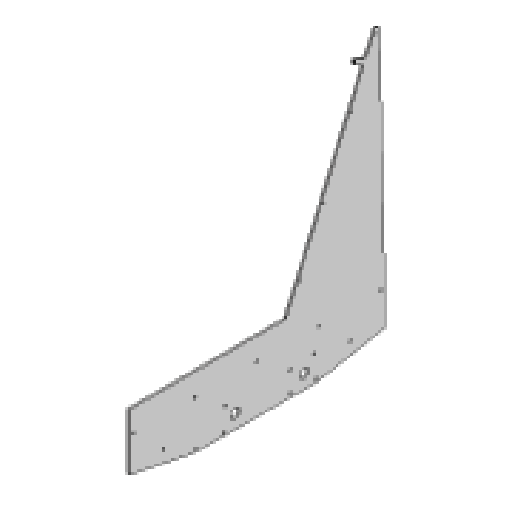
# Autodesk Inventor part: Outside Chassi Plate low 2.0
Saved by Autodesk Inventor 2023 (Build 270158000, 158)
## iProperties
Created: 2022-09-05
Part Number: Outside Chassi Plate low 2.0
Material: Generic
Document SubType Name: Modeling
Designer: deli
Density: 1 g/cm^3
Appearance: Default
Author: deli
Autodesk Inventor part; units mm, degrees
ref_plane "YZ Plane" through (0, 0, 0) normal (1, 0, 0) x (0, 1, 0)
ref_plane "XZ Plane" through (0, 0, 0) normal (0, 1, 0) x (-1, 0, 0)
ref_plane "XY Plane" through (0, 0, 0) normal (0, 0, 1) x (1, 0, 0)
sketch "Sketch1" plane through (0, 0, 0) normal (1, 0, 0) x (0, 1, 0)
  line L0 (-213.0456, 518.5703) -> (-297.1987, 518.5703)
  line L1 (-297.1987, 518.5703) -> (-316.9444, 421.9583)
  line L2 (-213.7388, 140.8703) -> (-297.8918, 140.8703)
  circle A0 centre (-289.0456, 468.5703) radius 2
  circle A1 centre (-289.0456, 468.5703) radius 48 construction
  arc A2 (-277.131, 467.8463) -> (-300.9481, 469.4724) centre (-289.0456, 468.5703) ccw construction
  circle A3 centre (-289.0456, 190.8703) radius 48 construction
  arc A4 (-300.901, 189.4801) -> (-277.1614, 191.9869) centre (-289.0456, 190.8703) ccw construction
  circle A5 centre (-289.0456, 190.8703) radius 2
  circle A6 centre (-296.2956, 362.3801) radius 7
  circle A7 centre (-296.2956, 259.5275) radius 7
  circle A8 centre (-296.2956, 362.3801) radius 18.75 construction
  circle A9 centre (-296.2956, 259.5275) radius 18.75 construction
  arc A10 (-308.9916, 363.3423) -> (-283.5867, 361.6078) centre (-296.2956, 362.3801) ccw construction
  arc A11 (-283.6191, 260.7186) -> (-308.9414, 258.0446) centre (-296.2956, 259.5275) ccw construction
  line L3 (-277.131, 467.8463) -> (-283.5867, 361.6078) construction
  line L4 (-308.9916, 363.3423) -> (-300.9481, 469.4724) construction
  line L5 (-283.6191, 260.7186) -> (-277.1614, 191.9869) construction
  line L6 (-300.901, 189.4801) -> (-308.9414, 258.0446) construction
  circle A12 centre (-281.2909, 280.4541) radius 2
  circle A13 centre (-311.3004, 280.4541) radius 2
  circle A14 centre (-312.0456, 379.4828) radius 2
  circle A15 centre (-312.0456, 242.4249) radius 2
  circle A16 centre (-278.1266, 245.0207) radius 2
  circle A17 centre (-246.0456, 513.5703) radius 2
  arc A18 (-317.0456, 229.9036) -> (-317.0456, 229.9036) centre (-294.2956, 229.9036) ccw
  line L7 (-317.0456, 242.4249) -> (-317.0456, 229.9036)
  arc A19 (-316.9444, 421.9583) -> (-317.0456, 420.9571) centre (-312.0456, 420.9571) ccw
  line L8 (-317.0456, 420.9571) -> (-317.0456, 229.9036)
  line L9 (-297.8918, 140.8703) -> (-316.9582, 241.4941)
  circle A20 centre (-278.6149, 377.4783) radius 2
  arc A21 (-317.0456, 242.4249) -> (-316.9582, 241.4941) centre (-312.0456, 242.4249) ccw
  circle A22 centre (-246.0456, 237.7953) radius 2
  line L10 (-213.0456, 518.5703) -> (-213.0456, 285.8158)
  circle A23 centre (-246.0456, 421.6453) radius 2
  circle A24 centre (-246.0456, 329.7203) radius 2
  circle A25 centre (-312.0456, 420.9571) radius 2
  circle A26 centre (-246.0456, 145.8703) radius 2
  line L11 (-179.9838, 271.6186) -> (-182.7458, 265.1866)
  line L12 (-182.7458, 265.1866) -> (92.9136, 146.8149)
  line L13 (92.9136, 146.8149) -> (95.6756, 153.2469)
  line L14 (628.6384, -183.2052) -> (619.1262, -197.2948) construction
  line L15 (-182.3379, 278.8085) -> (-189.0456, 263.1877) construction
  line L16 (-188.4024, 281.4126) -> (108.5747, 153.8869) construction
  line L17 (102.5102, 156.491) -> (95.8025, 140.8703) construction
  line L18 (95.8025, 140.8703) -> (-189.0456, 263.1877) construction
  line L19 (-184.6634, 286.0648) -> (-173.6371, 281.3299) construction
  line L20 (-173.6371, 281.3299) -> (-175.2154, 277.6545) construction
  line L21 (-175.2154, 277.6545) -> (-186.2417, 282.3893) construction
  line L22 (-186.2417, 282.3893) -> (-184.6634, 286.0648) construction
  line L23 (-185.4431, 288.3041) -> (-176.0707, 284.2795) construction
  line L24 (-178.4381, 278.7663) -> (-187.8106, 282.7909) construction
  line L25 (-176.0707, 284.2795) -> (-176.6626, 282.9012) construction
  line L26 (-178.4381, 278.7663) -> (-179.03, 277.388) construction
  line L27 (-176.6626, 282.9012) -> (-186.035, 286.9258) construction
  arc A27 (-185.4431, 288.3041) -> (-188.4024, 281.4126) centre (-186.9228, 284.8584) ccw construction
  arc A28 (-186.035, 286.9258) -> (-187.8106, 282.7909) centre (-186.9228, 284.8584) ccw construction
  line L28 (99.2023, 157.9115) -> (99.7941, 159.2898) construction
  line L29 (99.7941, 159.2898) -> (109.1666, 155.2652) construction
  arc A29 (109.1666, 155.2652) -> (110.9421, 159.4) centre (110.0544, 157.3326) ccw construction
  line L30 (110.9421, 159.4) -> (101.5697, 163.4247) construction
  line L31 (101.5697, 163.4247) -> (102.1616, 164.803) construction
  line L32 (102.1616, 164.803) -> (111.534, 160.7783) construction
  arc A30 (108.5747, 153.8869) -> (111.534, 160.7783) centre (110.0544, 157.3326) ccw construction
  line L33 (109.3733, 159.8016) -> (107.795, 156.1262) construction
  line L34 (107.795, 156.1262) -> (96.7686, 160.8611) construction
  line L35 (96.7686, 160.8611) -> (98.3469, 164.5365) construction
  line L36 (98.3469, 164.5365) -> (109.3733, 159.8016) construction
  line L37 (92.9136, 146.8149) -> (-213.7388, 140.8703)
  circle A31 centre (-174.4733, 265.4433) radius 1
  circle A32 centre (-91.7755, 229.9318) radius 1
  circle A33 centre (4.7053, 188.5017) radius 1
  circle A34 centre (87.4031, 152.9902) radius 1
  circle A35 centre (73.8024, 178.3411) radius 1.5
  arc A36 (76.559, 177.1574) -> (71.0458, 179.5248) centre (73.8024, 178.3411) ccw
  line L38 (71.0458, 179.5248) -> (67.2322, 170.6439)
  line L39 (76.559, 177.1574) -> (72.7454, 168.2765)
  line L40 (95.6756, 153.2469) -> (75.2424, 162.0212)
  line L41 (60.977, 168.147) -> (-213.0456, 285.8158)
  arc A37 (72.7454, 168.2765) -> (75.2424, 162.0212) centre (77.1215, 166.3973) ccw
  arc A38 (60.977, 168.147) -> (67.2322, 170.6439) centre (62.8562, 172.523) ccw
  circle A39 centre (73.8024, 178.3411) radius 6 construction
  circle A40 centre (-215.5456, 495.2703) radius 1.6
  circle A41 centre (-230.5456, 495.2703) radius 1.6
  circle A42 centre (-230.5456, 485.2703) radius 1.6
  circle A43 centre (-215.5456, 485.2703) radius 1.6
  circle A44 centre (-215.5456, 466.3703) radius 1.6
  circle A45 centre (-215.5456, 456.3703) radius 1.6
  circle A46 centre (-230.5456, 456.3703) radius 1.6
  circle A47 centre (-230.5456, 466.3703) radius 1.6
  line L42 (-215.5456, 495.2703) -> (-230.5456, 495.2703) construction
  line L43 (-230.5456, 495.2703) -> (-230.5456, 485.2703) construction
  line L44 (-230.5456, 485.2703) -> (-215.5456, 485.2703) construction
  line L45 (-215.5456, 485.2703) -> (-215.5456, 495.2703) construction
  line L46 (-215.5456, 456.3703) -> (-215.5456, 466.3703) construction
  line L47 (-215.5456, 466.3703) -> (-230.5456, 466.3703) construction
  line L48 (-230.5456, 466.3703) -> (-230.5456, 456.3703) construction
  line L49 (-230.5456, 456.3703) -> (-215.5456, 456.3703) construction
  point P0 (0, 0)
  point P1 (-317.0456, 242.4249)
  point P2 (-225.2933, 140.8703)
  dimension "d44" = 4
  dimension "d46" = 96
  dimension "d47" = 23.8732
  dimension "d48" = 96
  dimension "d49" = 4
  dimension "d51" = 23.8732
  dimension "d54" = 50
  dimension "d55" = 50
  dimension "d58" = 14
  dimension "d59" = 14
  dimension "d60" = 37.5
  dimension "d61" = 37.5
  dimension "d62" = 25.4648
  dimension "d63" = 25.4648
  dimension "d64" = 179.143
  dimension "d65" = 179.143
  dimension "d66" = 178.679
  dimension "d67" = 178.679
  dimension "d68" = 106.4344
  dimension "d70" = 69.0344
  dimension "d74" = 4
  dimension "d75" = 4
  dimension "d77" = 4
  dimension "d78" = 4
  dimension "d94" = 2.5
  dimension "d95" = 2.5
  dimension "d97" = 2.5
  dimension "d103" = 4
  dimension "d120" = 4
  dimension "d124" = 28
  dimension "d125" = 20.75
  dimension "d127" = 20.75
  dimension "d142" = 4
  dimension "d143" = 2.5
  dimension "d144" = 4
  dimension "d145" = 4
  dimension "d146" = 18
  dimension "d147" = 18
  dimension "d148" = 5
  dimension "d149" = 5
  dimension "d153" = 4
  dimension "d166" = 5
  dimension "d218" = 0
  dimension "d235" = 33
  dimension "d244" = 28
  dimension "d246" = 84.153
  dimension "d247" = 84.153
  dimension "d258" = 5
  dimension "d259" = 5
  dimension "d260" = 4
  dimension "d261" = 4
  dimension "d262" = 4
  dimension "d264" = 5
  dimension "d266" = 33
  dimension "d267" = 33
  dimension "d268" = 91.925
  dimension "d269" = 91.925
  dimension "d270" = 91.925
  dimension "d271" = 0
  dimension "d272" = 41.4743
  dimension "d277" = 5
  dimension "d296" = 33
  dimension "d297" = 7
  dimension "d317" = 0
  constraints: 100 end point, 48 centre point, 29 point on circle, 28 tangent, 23 perpendicular, 15 parallel, 12 equal radius, 10 coincident, 7 point on line, 4 collinear, 4 vertical, 3 concentric, 3 equal length
  measures "d44" diameter of A0
  measures "d46" diameter of A1
  measures "d47" diameter of A2
  measures "d48" diameter of A3
  measures "d49" diameter of A5
  measures "d51" diameter of A4
  measures "d54" distance from line of A0.centre L0
  measures "d55" distance from line of L2 A5.centre
  measures "d58" diameter of A6
  measures "d59" diameter of A7
  measures "d60" diameter of A8
  measures "d61" diameter of A9
  measures "d62" diameter of A10
  measures "d63" diameter of A11
  measures "d68" distance of L3.start L3.end
  measures "d70" distance of L5.start L5.end
  measures "d74" diameter of A14
  measures "d75" diameter of A13
  measures "d77" diameter of A12
  measures "d78" diameter of A16
  measures "d103" diameter of A17
  measures "d120" diameter of A15
  measures "d124" distance from line of A0.centre L7
  measures "d125" distance from line of L7 A6.centre
  measures "d127" distance from line of L7 A7.centre
  measures "d142" distance from line of L5 A16.centre
  measures "d144" distance from line of L3 A20.centre
  measures "d145" diameter of A20
  measures "d146" distance from line of A0.centre L1
  measures "d147" distance from line of L9 A3.centre
  measures "d148" radius of A19
  measures "d149" radius of A21
  measures "d153" diameter of A22
  measures "d166" distance from line of L8 A14.centre
  measures "d218" horizontal distance of A0.centre A5.centre
  measures "d235" distance from line of L10 A17.centre
  measures "d244" distance edge to line of A1 L10
  measures "d246" distance of L2.start L2.end
  measures "d247" distance of L0.start L0.end
  measures "d260" diameter of A23
  measures "d261" diameter of A24
  measures "d262" diameter of A25
  measures "d264" distance from line of L8 A25.centre
  measures "d266" distance from line of L10 A23.centre
  measures "d267" distance from line of L10 A24.centre
  measures "d268" distance of A23.centre A17.centre
  measures "d269" distance of A24.centre A23.centre
  measures "d270" distance of A22.centre A24.centre
  measures "d271" distance of A25.centre A19.centre
  measures "d272" distance of A14.centre A25.centre
  measures "d277" distance from line of L2 A26.centre
  measures "d296" distance from line of L10 A22.centre
  measures "d297" distance of L11.start L11.end
  measures "d317" horizontal distance of A26.centre A22.centre
extrude "Extrusion1" add sketch "Sketch1" along normal blind 3.175 contours L10 L41 L11 L12 L37 L2 L9 A18 A16 A7 A15 A21 L8 A19 L1 L0 | L41 A38 L38 A36 L39 A37 L40 L13 L12 L11 | A18 A15 A7 A16 L9
thread "Thread1" size "M2x0.4" class "6H" standard "ANSI Metric M Profile" full length
thread "Thread2" size "M2x0.4" class "6H" standard "ANSI Metric M Profile" full length
thread "Thread3" size "M2x0.4" class "6H" standard "ANSI Metric M Profile" full length
fillet "Fillet1" radius 2 2 edges at (1.5875, 95.6756, 153.2469) (1.5875, -213.0456, 285.8158)
thread "Thread4" size "M2x0.4" class "6H" standard "ANSI Metric M Profile" full length
body "Solid1"
